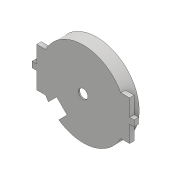
# Autodesk Inventor part: SnackClock_exterior_final
Saved by Autodesk Inventor 2018 (Build 220112000, 112)
## iProperties
Created: 2018-02-19
Part Number: SnackClock_exterior_final
Material: Generic
Document SubType Name: Modeling
Designer: Katrina
Density: 1 g/cm^3
Appearance: Default
Mass: 16.0833 g
Surface Area: 143.662 cm^2
Volume: 16.0833 cm^3
Author: Katrina
Autodesk Inventor part; units mm, degrees
ref_plane "YZ Plane" through (0, 0, 0) normal (1, 0, 0) x (0, 1, 0)
ref_plane "XZ Plane" through (0, 0, 0) normal (0, 1, 0) x (-1, 0, 0)
ref_plane "XY Plane" through (0, 0, 0) normal (0, 0, 1) x (1, 0, 0)
sketch "Sketch1" plane through (0, 0, 0) normal (0, 1, 0) x (-1, 0, 0)
  circle A0 centre (0, 0) radius 37.5
  dimension "d0" = 75
  constraints: 1 centre point, 1 coincident
  measures "d0" diameter of A0
extrude "Extrusion1" add sketch "Sketch1" along normal blind 12
sketch "Sketch3" plane through (0, 0, 0) normal (0, -1, 0) x (1, 0, 0)
  line L0 (41, 17.5) -> (-41, 17.5)
  line L1 (-41, 17.5) -> (-41, -17.5)
  line L2 (-41, -17.5) -> (41, -17.5)
  line L3 (41, -17.5) -> (41, 17.5)
  point P0 (0, 0)
  point P1 (41, 0)
  point P2 (0, -17.5)
  dimension "d6" = 82
  dimension "d7" = 35
  constraints: 8 end point, 2 midpoint, 2 parallel, 1 horizontal, 1 horizontal alignment, 1 perpendicular, 1 vertical alignment
  measures "d6" distance of L2.end L1.end
  measures "d7" distance of L1.end L0.end
extrude "Extrusion3" add sketch "Sketch3" against normal blind 4
sketch "Sketch4" plane through (0, 0, 0) normal (0, -1, 0) x (1, 0, 0)
  line L0 (-45, -2.625) -> (45, -2.625)
  line L1 (45, -2.625) -> (45, 2.625)
  line L2 (45, 2.625) -> (-45, 2.625)
  line L3 (-45, 2.625) -> (-45, -2.625)
  point P0 (0, 0)
  point P1 (-45, 0)
  point P2 (0, 2.625)
  dimension "d10" = 90
  dimension "d11" = 5.25
  constraints: 8 end point, 2 midpoint, 2 parallel, 1 horizontal, 1 horizontal alignment, 1 perpendicular, 1 vertical alignment
  measures "d10" distance of L2.end L1.end
  measures "d11" distance of L1.end L0.end
extrude "Extrusion4" add sketch "Sketch4" against normal blind 4
sketch "Sketch2" plane through (0, 12, 0) normal (0, 1, 0) x (1, 0, 0)
  circle A0 centre (0, 0) radius 33
  dimension "d3" = 66
  constraints: 1 centre point, 1 coincident
  measures "d3" diameter of A0
extrude "Extrusion2" cut sketch "Sketch2" against normal blind 11
sketch "Sketch5" plane through (0, 1, 0) normal (0, 1, 0) x (1, 0, 0)
  circle A0 centre (0, 0) radius 4.1
  dimension "d14" = 8.2
  constraints: 1 centre point, 1 coincident
  measures "d14" diameter of A0
extrude "Extrusion5" cut sketch "Sketch5" against normal through all
sketch "Sketch6" plane through (0, 12, 0) normal (0, 1, 0) x (1, 0, 0)
  line L0 (-23.4141, 14.0625) -> (-31.1923, 21.8407)
  line L1 (-31.1923, 21.8407) -> (-21.9999, 31.0331)
  line L2 (-21.9999, 31.0331) -> (-14.2217, 23.2549)
  line L3 (-14.2217, 23.2549) -> (-23.4141, 14.0625)
  line L4 (0, 0) -> (-32.7126, 0) construction
  line L5 (0, 0) -> (0, 33) construction
  circle A0 centre (0, 0) radius 33 construction
  circle A1 centre (0, 0) radius 37.5 construction
  dimension "d17" = 11
  dimension "d18" = 13
  constraints: 12 end point, 2 parallel, 1 horizontal, 1 perpendicular, 1 tangent, 1 vertical, 1 vertical alignment, 1 other
  measures "d17" distance of L1.end L2.end
  measures "d18" distance of L0.end L1.end
extrude "Extrusion6" cut sketch "Sketch6" against normal through all
body "Solid1"
